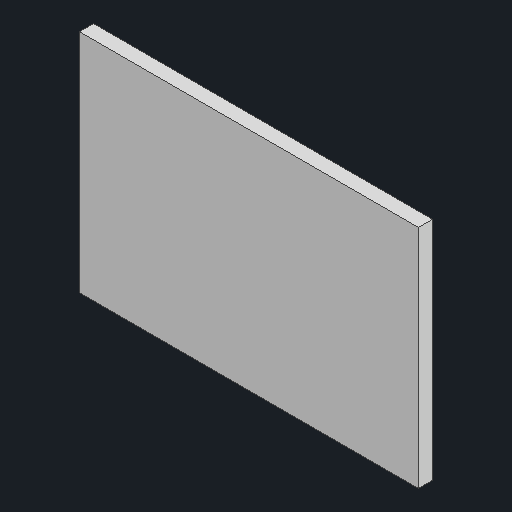
# Autodesk Inventor part: FLAT-PL
Saved by Autodesk Inventor 2027 (Build 310192000, 192)
## iProperties
Created: 2026-04-27
Part Number: FLAT-PL
Material: Generic
Description: PL 1/4 X 4 X 6
Document SubType Name: Modeling
Designer: mstri
Density: 1 g/cm^3
Appearance: Default
MCP_RevitFamily: STEEL_PLATE 1-4 x 4 x Length
MCP_RevitElemId: 4628909
MANUFACTURE_COMPONENT: PLATE ASSEMBLY COMPONENT RAW CONSUMABLE
CONTROL_MARK: FLAT-PL
SORTING_ORDER: 504
MCP_MIN_TEST: ok
IDENTITY_DESCRIPTION_SHORT: FLAT-PL
MCP_TEST_A: A
MCP_TEST_B: B
IDENTITY_DESCRIPTION: PL 1/4" X 4" X (SCHEDULED LENGTH)
DIM_LENGTH: 0.5
QTY_MULTIPLIER: 1
ASSEMBLY_COMPONENT: 1
MANUFACTURER_PLANT_ID: Plant ID B (edit)
MANUFACTURER_PLANT_DESCRIPTION: Plant Description B (edit)
DIM_LENGTH_IN: 6
MCP_DIM_SOURCE_UNITS: Revit length doubles in feet
Author: mstri
Autodesk Inventor part; units mm, degrees
ref_plane "YZ Plane" through (0, 0, 0) normal (1, 0, 0) x (0, 1, 0)
ref_plane "XZ Plane" through (0, 0, 0) normal (0, 1, 0) x (-1, 0, 0)
ref_plane "XY Plane" through (0, 0, 0) normal (0, 0, 1) x (1, 0, 0)
sketch "Sketch6" plane through (0, 0, 0) normal (0, 0, 1) x (1, 0, 0)
  line L0 (-76.2, -50.8) -> (76.2, -50.8)
  line L1 (76.2, -50.8) -> (76.2, 50.8)
  line L2 (76.2, 50.8) -> (-76.2, 50.8)
  line L3 (-76.2, 50.8) -> (-76.2, -50.8)
  constraints: 8 end point, 2 parallel, 1 horizontal, 1 perpendicular
extrude "P351_PlateBody" add sketch "Sketch6" along normal blind 6.35
equation "\"PlateLength\" = 152.4"
equation "\"PlateWidth\" = 101.6"
equation "\"PlateThickness\" = 6.35"
equation "\"DIM_LENGTH\" = 152.4"
body "Solid6"
